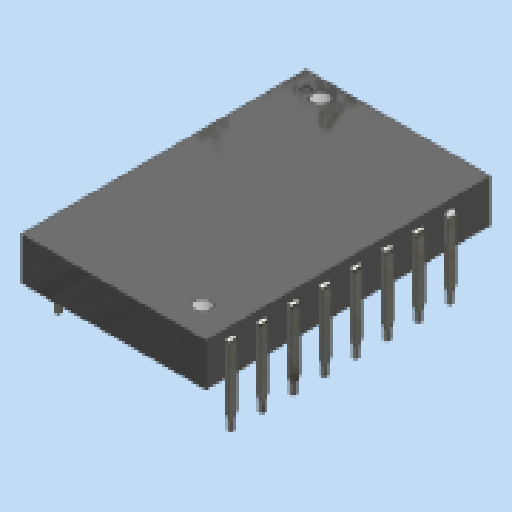
# Autodesk Inventor part: PMW3360_sensor
Saved by Autodesk Inventor 2024 (Build 280153000, 153)
## iProperties
Created: 2025-05-06
Part Number: PMW3360_sensor
Material: Generic
Document SubType Name: Modeling
Designer: XxPan
Density: 1 g/cm^3
Appearance: Default
Author: XxPan
Autodesk Inventor part; units mm, degrees
ref_plane "YZ Plane" through (0, 0, 0) normal (1, 0, 0) x (0, 1, 0)
ref_plane "XZ Plane" through (0, 0, 0) normal (0, 1, 0) x (-1, 0, 0)
ref_plane "XY Plane" through (0, 0, 0) normal (0, 0, 1) x (1, 0, 0)
sketch "Sketch1" plane through (0, 0, 0) normal (0, 1, 0) x (-1, 0, 0)
  line L0 (5.25, 8.1) -> (-5.25, 8.1)
  line L1 (-5.25, 8.1) -> (-5.25, -8.1)
  line L2 (-5.25, -8.1) -> (5.25, -8.1)
  line L3 (5.25, -8.1) -> (5.25, 8.1)
  line L4 (7.35, 0) -> (-7.35, 0) construction
  line L5 (0, -11.34) -> (0, 11.34) construction
  point P0 (0, 0)
  dimension "d0" = 10.5
  dimension "d1" = 16.2
  constraints: 8 end point, 2 parallel, 1 horizontal, 1 perpendicular, 2 other
  measures "d0" distance of L2.end L1.end
  measures "d1" distance of L1.end L0.end
extrude "Extrusion1" add sketch "Sketch1" along normal blind 2.41
sketch "Sketch2" plane through (0, 2.41, 0) normal (0, 1, 0) x (1, 0, 0)
  circle A0 centre (-4.25, 7.1) radius 0.25
  line L0 (-5.25, 8.1) -> (-5.25, -8.1) projected
  line L1 (5.25, 8.1) -> (-5.25, 8.1) projected
  point P0 (0, 0)
  dimension "d4" = 0.5
  dimension "d5" = 1
  dimension "d6" = 1
  constraints: 1 centre point
  measures "d4" diameter of A0
  measures "d5" distance from line of L0 A0.centre
  measures "d6" distance from line of L1 A0.centre
extrude "Extrusion2" cut sketch "Sketch2" against normal blind 0.1
sketch "Sketch6" plane through (0, 2.41, 0) normal (0, 1, 0) x (1, 0, 0)
  circle A0 centre (-3.415, 7.1) radius 0.45
  circle A1 centre (3.415, -6.44) radius 0.45
  line L0 (5.25, 8.1) -> (-5.25, 8.1) projected
  point P0 (0, 0)
  dimension "d47" = 0.9
  dimension "d48" = 0.9
  dimension "d49" = 6.83
  dimension "d50" = 3.415
  dimension "d51" = 0.55
  dimension "d52" = 13.54
  constraints: 2 centre point
  measures "d47" diameter of A0
  measures "d48" diameter of A1
  measures "d49" horizontal distance of A1.centre A0.centre
  measures "d50" horizontal distance of point (0, 0) A0.centre
  measures "d51" distance edge to line of A0 L0
  measures "d52" vertical distance of A1.centre A0.centre
extrude "Extrusion6" cut sketch "Sketch6" against normal through all
sketch "Sketch5" plane through (0, 0, 0) normal (0, -1, 0) x (1, 0, 0)
  circle A0 centre (0, 0) radius 2
  circle A1 centre (0, 0) radius 0.4
  dimension "d40" = 4
  dimension "d41" = 0.8
  constraints: 2 centre point, 2 coincident
  measures "d40" diameter of A0
  measures "d41" diameter of A1
extrude "Extrusion5" add sketch "Sketch5" along normal blind 1.7
fillet "Fillet1" radius 0.5 1 edges at (-2, -1.7, 0)
sketch "Sketch3" plane through (-5.25, 0, -8.1) normal (-1, 0, 0) x (0, 0, 1)
  line L0 (1.27, 1.91) -> (1.77, 1.91)
  line L1 (1.77, 1.91) -> (1.77, -1.7)
  line L2 (16.2, 0) -> (0, 0) construction
  line L3 (1.77, -1.7) -> (1.645, -2)
  line L4 (1.645, -2) -> (1.645, -2.6)
  line L5 (1.645, -2.6) -> (1.395, -2.6)
  line L6 (1.395, -2.6) -> (1.395, -2)
  line L7 (1.395, -2) -> (1.27, -1.7)
  line L8 (1.27, -1.7) -> (1.27, 1.91)
  line L9 (0, 2.41) -> (16.2, 2.41) construction
  line L10 (0, 0) -> (0, 2.41) construction
  point P0 (8.1, 0)
  point P1 (1.52, 1.91)
  dimension "d9" = 0.5
  dimension "d10" = 0.25
  dimension "d11" = 1.91
  dimension "d12" = 4.11
  dimension "d13" = 4.51
  dimension "d14" = 0.9
  dimension "d15" = 0.3
  dimension "d16" = 1.52
  dimension "d17" = 0.125
  constraints: 16 end point, 3 perpendicular, 2 horizontal alignment, 2 parallel, 1 horizontal, 1 midpoint
  measures "d9" distance between parallel lines of L1 L8
  measures "d10" distance of L4.end L5.end
  measures "d11" distance between parallel lines of L2 L0
  measures "d12" distance from line of L7.end L9
  measures "d13" distance between parallel lines of L5 L0
  measures "d14" distance from line of L7.end L5
  measures "d15" vertical distance of L6.end L7.end
  measures "d16" distance from line of point (1.52, 1.91) L10
  measures "d17" distance between parallel lines of L8 L6
extrude "Extrusion3" add sketch "Sketch3" along normal blind 0.2
sketch "Sketch4" plane through (5.25, 0, 8.1) normal (1, 0, 0) x (0, 0, -1)
  line L0 (13.54, 1.91) -> (14.04, 1.91)
  line L1 (14.04, 1.91) -> (14.04, -1.7)
  line L2 (14.04, -1.7) -> (13.915, -2)
  line L3 (13.915, -2) -> (13.915, -2.6)
  line L4 (13.915, -2.6) -> (13.665, -2.6)
  line L5 (13.665, -2.6) -> (13.665, -2)
  line L6 (13.665, -2) -> (13.54, -1.7)
  line L7 (13.54, -1.7) -> (13.54, 1.91)
  line L8 (0, 2.41) -> (16.2, 2.41) construction
  line L9 (0, 0) -> (16.2, 0) construction
  line L10 (14.93, 1.91) -> (14.43, 1.91) projected
  point P0 (8.1, 0)
  point P1 (12.5997, 0.5868)
  point P2 (13.79, 1.91)
  point P3 (14.68, 1.91)
  dimension "d20" = 0.5
  dimension "d21" = 0.25
  dimension "d24" = 4.51
  dimension "d25" = 0.9
  dimension "d26" = 0.3
  dimension "d28" = 0.125
  dimension "d29" = 4.11
  dimension "d30" = 1.91
  dimension "d31" = 0.89
  constraints: 16 end point, 2 horizontal alignment, 2 midpoint, 2 parallel, 2 perpendicular, 1 horizontal
  measures "d20" distance between parallel lines of L1 L7
  measures "d21" distance of L3.end L4.end
  measures "d24" distance between parallel lines of L4 L0
  measures "d25" distance from line of L6.end L4
  measures "d26" vertical distance of L5.end L6.end
  measures "d28" distance between parallel lines of L7 L5
  measures "d29" distance from line of L8 L6.end
  measures "d30" distance between parallel lines of L9 L0
  measures "d31" distance of point (14.68, 1.91) point (13.79, 1.91)
extrude "Extrusion4" add sketch "Sketch4" along normal blind 0.2
fillet "Fillet2" radius 0.2 1 edges at (-5.45, 1.91, -6.58)
fillet "Fillet3" radius 0.2 1 edges at (5.45, 1.91, -5.69)
pattern_linear "Rectangular Pattern1" count 8 spacing 1.78 along (0, 0, 1) of "Extrusion3", "Fillet2"
pattern_linear "Rectangular Pattern2" count 8 spacing 1.78 along (0, 0, 1) of "Extrusion4", "Fillet3"
equation "\"d50\" = 0.5 * d49"
equation "\"d15\" = 0.333333 * d14"
equation "\"d17\" = -0.5 * d10 + 0.5 * d9"
equation "\"d26\" = 0.333333 * d25"
equation "\"d28\" = -0.5 * d21 + 0.5 * d20"
body "Solid1"
